Autodesk Fusion 360 part; units mm, degrees
(part 3 of 25)
  arc A722 (33.6042, 52.4764) -> (33.6042, 52.5272) centre (33.6042, 52.5018) ccw
  arc A723 (33.5788, 54.8259) -> (33.6296, 54.8259) centre (33.6042, 54.8259) ccw
  arc A724 (32.4358, 52.5272) -> (32.4358, 52.4764) centre (32.4358, 52.5018) ccw
  arc A725 (32.9297, 55.2154) -> (32.9805, 55.2154) centre (32.9551, 55.2154) ccw
  arc A726 (41.2242, 53.9821) -> (41.2242, 54.0329) centre (41.2242, 54.0075) ccw
  arc A727 (33.5788, 55.1504) -> (33.6296, 55.1504) centre (33.6042, 55.1504) ccw
  arc A728 (54.4034, 1.5804) -> (54.4542, 1.5804) centre (54.4288, 1.5804) ccw
  arc A729 (32.9297, 54.9557) -> (32.9805, 54.9557) centre (32.9551, 54.9557) ccw
  arc A730 (32.4104, 52.8264) -> (32.4612, 52.8264) centre (32.4358, 52.8264) ccw
  arc A731 (34.9758, 52.5272) -> (34.9758, 52.4764) centre (34.9758, 52.5018) ccw
  arc A732 (32.4612, 55.2154) -> (32.4104, 55.2154) centre (32.4358, 55.2154) ccw
  arc A733 (40.64, 54.8005) -> (40.64, 54.8513) centre (40.64, 54.8259) ccw
  arc A734 (29.7942, 28.6145) -> (29.7942, 28.6653) centre (29.7942, 28.6399) ccw
  arc A735 (32.7604, 53.1255) -> (32.7604, 53.1763) centre (32.7604, 53.1509) ccw
  arc A736 (32.6756, 53.667) -> (32.7153, 53.6988) centre (32.6955, 53.6829) ccw
  arc A737 (32.4358, 54.0329) -> (32.4358, 53.9821) centre (32.4358, 54.0075) ccw
  arc A738 (41.2496, 54.332) -> (41.1988, 54.332) centre (41.2242, 54.332) ccw
  arc A739 (40.0558, 55.1504) -> (40.2181, 54.9233) centre (40.2959, 55.1504) ccw
  arc A740 (33.6296, 52.8264) -> (33.5788, 52.8264) centre (33.6042, 52.8264) ccw
  line L231 (32.6954, 53.6829) -> (32.4358, 54.0075)
  arc A741 (40.2181, 54.9233) -> (40.64, 54.8259) centre (40.6401, 55.7886) ccw
  arc A742 (41.1988, 53.6829) -> (41.2496, 53.6829) centre (41.2242, 53.6829) ccw
  arc A743 (26.1112, 29.924) -> (26.0604, 29.924) centre (26.0858, 29.924) ccw
  arc A744 (32.7604, 53.1509) -> (32.4358, 52.8264) centre (32.7604, 52.8263) ccw
  arc A745 (33.6042, 52.8264) -> (33.2796, 53.1509) centre (33.2796, 52.8263) ccw
  arc A746 (40.2292, 54.9461) -> (40.2069, 54.9004) centre (40.2181, 54.9233) ccw
  arc A747 (33.6042, 53.9821) -> (33.6042, 54.0329) centre (33.6042, 54.0075) ccw
  arc A748 (32.9805, 55.2154) -> (32.9297, 55.2154) centre (32.9551, 55.2154) ccw
  arc A749 (33.5788, 53.6829) -> (33.6296, 53.6829) centre (33.6042, 53.6829) ccw
  line L232 (32.9551, 55.2154) -> (32.9551, 54.9557)
  line L233 (36.1442, 52.8264) -> (36.1442, 52.5018)
  line L234 (34.9758, 52.5018) -> (34.9758, 52.8264)
  arc A750 (36.1696, 52.8264) -> (36.1188, 52.8264) centre (36.1442, 52.8264) ccw
  arc A751 (36.1277, 54.8065) -> (36.1607, 54.8452) centre (36.1442, 54.8258) ccw
  arc A752 (37.8404, 53.1509) -> (37.5158, 52.8264) centre (37.8404, 52.8263) ccw
  arc A753 (36.1442, 52.8264) -> (35.8196, 53.1509) centre (35.8196, 52.8263) ccw
  arc A754 (34.9956, 54.0233) -> (34.956, 53.9916) centre (34.9758, 54.0074) ccw
  arc A755 (38.3596, 53.1763) -> (38.3596, 53.1255) centre (38.3596, 53.1509) ccw
  arc A756 (35.3004, 53.1509) -> (34.9758, 52.8264) centre (35.3004, 52.8263) ccw
  arc A757 (38.3596, 53.1255) -> (38.3596, 53.1763) centre (38.3596, 53.1509) ccw
  arc A758 (38.6842, 53.9821) -> (38.6842, 54.0329) centre (38.6842, 54.0075) ccw
  arc A759 (34.9504, 52.8264) -> (35.0012, 52.8264) centre (34.9758, 52.8264) ccw
  line L235 (35.4951, 55.3776) -> (36.1442, 54.8259)
  line L236 (37.7754, 54.8259) -> (37.5158, 55.1504)
  line L237 (35.3004, 53.1509) -> (35.8196, 53.1509)
  line L238 (37.5158, 52.5018) -> (37.5158, 52.8264)
  arc A760 (35.2679, 55.5004) -> (35.2679, 55.4496) centre (35.2679, 55.475) ccw
  arc A761 (36.1442, 53.9821) -> (36.1442, 54.0329) centre (36.1442, 54.0075) ccw
  arc A762 (37.5412, 52.8264) -> (37.4904, 52.8264) centre (37.5158, 52.8264) ccw
  line L239 (36.1442, 53.6829) -> (36.1442, 54.332)
  arc A763 (35.3004, 53.1763) -> (35.3004, 53.1255) centre (35.3004, 53.1509) ccw
  arc A764 (36.1188, 52.5018) -> (36.1696, 52.5018) centre (36.1442, 52.5018) ccw
  arc A765 (37.4904, 52.8264) -> (37.5412, 52.8264) centre (37.5158, 52.8264) ccw
  line L240 (38.6842, 52.8264) -> (38.6842, 52.5018)
  arc A766 (35.5115, 55.397) -> (35.4786, 55.3583) centre (35.495, 55.3777) ccw
  arc A767 (37.4904, 52.5018) -> (37.5412, 52.5018) centre (37.5158, 52.5018) ccw
  arc A768 (38.6588, 52.5018) -> (38.7096, 52.5018) centre (38.6842, 52.5018) ccw
  line L241 (37.5158, 54.0075) -> (38.6842, 54.0075)
  arc A769 (37.8404, 53.1255) -> (37.8404, 53.1763) centre (37.8404, 53.1509) ccw
  arc A770 (35.4951, 55.3776) -> (35.2679, 55.475) centre (35.2679, 55.1613) ccw
  line L242 (35.2354, 53.6829) -> (34.9758, 54.0075)
  arc A771 (38.6842, 52.4764) -> (38.6842, 52.5272) centre (38.6842, 52.5018) ccw
  arc A772 (37.8404, 53.1763) -> (37.8404, 53.1255) centre (37.8404, 53.1509) ccw
  arc A773 (35.8196, 53.1255) -> (35.8196, 53.1763) centre (35.8196, 53.1509) ccw
  arc A774 (36.1696, 54.332) -> (36.1188, 54.332) centre (36.1442, 54.332) ccw
  arc A775 (34.9504, 55.1829) -> (35.0012, 55.1829) centre (34.9758, 55.1829) ccw
  arc A776 (34.9758, 55.1829) -> (35.2354, 54.8259) centre (35.351, 55.1829) ccw
  arc A777 (34.9504, 52.5018) -> (35.0012, 52.5018) centre (34.9758, 52.5018) ccw
  line L243 (36.1442, 54.8259) -> (36.1442, 55.475)
  arc A778 (35.8196, 53.1763) -> (35.8196, 53.1255) centre (35.8196, 53.1509) ccw
  arc A779 (36.1188, 54.8259) -> (36.1696, 54.8259) centre (36.1442, 54.8259) ccw
  arc A780 (34.9758, 54.0329) -> (34.9758, 53.9821) centre (34.9758, 54.0075) ccw
  line L244 (34.9758, 54.0075) -> (36.1442, 54.0075)
  arc A781 (35.2679, 55.4496) -> (35.2679, 55.5004) centre (35.2679, 55.475) ccw
  arc A782 (36.1696, 55.475) -> (36.1188, 55.475) centre (36.1442, 55.475) ccw
  line L245 (38.6842, 52.5018) -> (37.5158, 52.5018)
  arc A783 (35.0012, 55.1829) -> (34.9504, 55.1829) centre (34.9758, 55.1829) ccw
  arc A784 (36.1188, 52.8264) -> (36.1696, 52.8264) centre (36.1442, 52.8264) ccw
  arc A785 (35.0012, 52.8264) -> (34.9504, 52.8264) centre (34.9758, 52.8264) ccw
  arc A786 (35.3004, 53.1255) -> (35.3004, 53.1763) centre (35.3004, 53.1509) ccw
  arc A787 (35.2679, 55.475) -> (34.9758, 55.1829) centre (35.2679, 55.1829) ccw
  arc A788 (35.4767, 55.3601) -> (35.5135, 55.3952) centre (35.4951, 55.3777) ccw
  arc A789 (37.5158, 52.5272) -> (37.5158, 52.4764) centre (37.5158, 52.5018) ccw
  arc A790 (36.1188, 53.6829) -> (36.1696, 53.6829) centre (36.1442, 53.6829) ccw
  line L246 (37.8404, 53.1509) -> (38.3596, 53.1509)
  arc A791 (38.7096, 52.8264) -> (38.6588, 52.8264) centre (38.6842, 52.8264) ccw
  arc A792 (38.6588, 52.8264) -> (38.7096, 52.8264) centre (38.6842, 52.8264) ccw
  arc A793 (38.6842, 52.8264) -> (38.3596, 53.1509) centre (38.3596, 52.8263) ccw
  arc A794 (37.5356, 54.0233) -> (37.496, 53.9916) centre (37.5158, 54.0074) ccw
  line L247 (37.7754, 53.6829) -> (37.5158, 54.0075)
  arc A795 (37.7556, 53.667) -> (37.7953, 53.6988) centre (37.7754, 53.6829) ccw
  arc A796 (35.2156, 53.667) -> (35.2553, 53.6988) centre (35.2355, 53.6829) ccw
  arc A797 (38.6588, 53.6829) -> (38.7096, 53.6829) centre (38.6842, 53.6829) ccw
  arc A798 (35.2276, 54.8017) -> (35.2433, 54.8501) centre (35.2355, 54.8259) ccw
  line L248 (37.5158, 55.1504) -> (38.6842, 55.1504)
  arc A799 (37.5158, 55.1758) -> (37.5158, 55.125) centre (37.5158, 55.1504) ccw
  arc A800 (38.7096, 54.332) -> (38.6588, 54.332) centre (38.6842, 54.332) ccw
  arc A801 (37.5356, 55.1663) -> (37.496, 55.1346) centre (37.5158, 55.1504) ccw
  arc A802 (37.7556, 54.81) -> (37.7953, 54.8418) centre (37.7754, 54.8259) ccw
  arc A803 (38.6842, 55.125) -> (38.6842, 55.1758) centre (38.6842, 55.1504) ccw
  line L249 (38.6842, 53.6829) -> (38.6842, 54.332)
  arc A804 (37.5158, 54.0329) -> (37.5158, 53.9821) centre (37.5158, 54.0075) ccw
  line L250 (41.2242, 52.5018) -> (40.0558, 52.5018)
  arc A805 (33.6804, 29.5557) -> (33.7312, 29.5557) centre (33.7058, 29.5557) ccw
  arc A806 (40.3804, 53.1255) -> (40.3804, 53.1763) centre (40.3804, 53.1509) ccw
  arc A807 (33.9979, 29.8478) -> (33.7058, 29.5557) centre (33.9979, 29.5557) ccw
  arc A808 (34.5567, 28.0882) -> (34.6075, 28.0882) centre (34.5821, 28.0882) ccw
  line L251 (38.6842, 54.8259) -> (38.6842, 55.475)
  line L252 (37.4974, 2.4892) -> (37.4974, 1.3208)
  arc A809 (38.6588, 54.8259) -> (38.7096, 54.8259) centre (38.6842, 54.8259) ccw
  arc A810 (40.0812, 52.8264) -> (40.0304, 52.8264) centre (40.0558, 52.8264) ccw
  arc A811 (41.2242, 52.4764) -> (41.2242, 52.5272) centre (41.2242, 52.5018) ccw
  arc A812 (40.3804, 53.1763) -> (40.3804, 53.1255) centre (40.3804, 53.1509) ccw
  line L253 (40.3804, 53.1509) -> (40.8996, 53.1509)
  line L254 (41.2242, 52.8264) -> (41.2242, 52.5018)
  arc A813 (34.6075, 28.6724) -> (34.5567, 28.6724) centre (34.5821, 28.6724) ccw
  arc A814 (40.0304, 52.8264) -> (40.0812, 52.8264) centre (40.0558, 52.8264) ccw
  arc A815 (40.3804, 53.1509) -> (40.0558, 52.8264) centre (40.3804, 52.8263) ccw
  arc A816 (41.2242, 52.8264) -> (40.8996, 53.1509) centre (40.8996, 52.8263) ccw
  arc A817 (37.157, 2.2494) -> (37.1888, 2.2097) centre (37.1729, 2.2296) ccw
  arc A818 (41.1988, 52.8264) -> (41.2496, 52.8264) centre (41.2242, 52.8264) ccw
  arc A819 (37.472, 1.3208) -> (37.5228, 1.3208) centre (37.4974, 1.3208) ccw
  line L255 (37.1729, 2.2296) -> (37.4974, 2.4892)
  arc A820 (37.1729, 1.3462) -> (37.1729, 1.2954) centre (37.1729, 1.3208) ccw
  line L256 (38.9636, 2.4892) -> (38.9636, 1.6454)
  arc A821 (34.8577, 29.1794) -> (34.8907, 29.2181) centre (34.8742, 29.1988) ccw
  arc A822 (37.5133, 2.4694) -> (37.4816, 2.509) centre (37.4975, 2.4892) ccw
  arc A823 (37.5228, 2.4892) -> (37.472, 2.4892) centre (37.4974, 2.4892) ccw
  line L257 (37.1729, 1.3208) -> (37.822, 1.3208)
  line L258 (40.0558, 52.5018) -> (40.0558, 52.8264)
  arc A824 (40.0304, 52.5018) -> (40.0812, 52.5018) centre (40.0558, 52.5018) ccw
  arc A825 (40.8996, 53.1763) -> (40.8996, 53.1255) centre (40.8996, 53.1509) ccw
  arc A826 (40.0558, 52.5272) -> (40.0558, 52.4764) centre (40.0558, 52.5018) ccw
  arc A827 (38.7096, 55.475) -> (38.6588, 55.475) centre (38.6842, 55.475) ccw
  arc A828 (40.8996, 53.1255) -> (40.8996, 53.1763) centre (40.8996, 53.1509) ccw
  arc A829 (33.9979, 29.8732) -> (33.9979, 29.8224) centre (33.9979, 29.8478) ccw
  arc A830 (38.9382, 1.6454) -> (38.989, 1.6454) centre (38.9636, 1.6454) ccw
  arc A831 (39.6381, 2.4892) -> (39.5873, 2.4892) centre (39.6127, 2.4892) ccw
  line L259 (39.6127, 1.6454) -> (39.6127, 2.4892)
  line L260 (44.8779, 1.3208) -> (44.6182, 1.8401)
  arc A832 (41.33, 2.5146) -> (41.33, 2.4638) centre (41.33, 2.4892) ccw
  arc A833 (45.3263, 1.4831) -> (45.7157, 1.3208) centre (45.7158, 1.8692) ccw
  arc A834 (41.5897, 2.4638) -> (41.5897, 2.5146) centre (41.5897, 2.4892) ccw
  line L261 (41.4598, 2.4892) -> (41.4598, 1.3208)
  line L262 (41.33, 2.4892) -> (41.5897, 2.4892)
  arc A835 (41.33, 1.3462) -> (41.33, 1.2954) centre (41.33, 1.3208) ccw
  arc A836 (40.2082, 2.4892) -> (40.1574, 2.4892) centre (40.1828, 2.4892) ccw
  arc A837 (37.822, 1.2954) -> (37.822, 1.3462) centre (37.822, 1.3208) ccw
  arc A838 (40.1574, 1.3208) -> (40.2082, 1.3208) centre (40.1828, 1.3208) ccw
  arc A839 (40.8065, 1.3208) -> (40.8573, 1.3208) centre (40.8319, 1.3208) ccw
  line L263 (42.3742, 1.3208) -> (42.7637, 2.4892)
  line L264 (43.233, 2.4892) -> (43.7523, 2.4892)
  line L265 (43.7523, 1.3208) -> (43.233, 1.3208)
  arc A840 (42.3501, 1.3288) -> (42.3983, 1.3128) centre (42.3742, 1.3208) ccw
  arc A841 (43.6225, 1.9445) -> (43.6225, 1.9953) centre (43.6225, 1.9699) ccw
  arc A842 (44.2033, 1.3208) -> (44.2541, 1.3208) centre (44.2287, 1.3208) ccw
  arc A843 (44.2287, 2.5146) -> (44.2287, 2.4638) centre (44.2287, 2.4892) ccw
  arc A844 (41.4852, 2.4892) -> (41.4344, 2.4892) centre (41.4598, 2.4892) ccw
  line L266 (41.9848, 2.4892) -> (42.3742, 1.3208)
  line L267 (40.1828, 2.4892) -> (40.8319, 1.3208)
  arc A845 (38.9636, 1.6454) -> (39.6127, 1.6454) centre (39.2881, 1.6454) ccw
  arc A846 (40.8097, 1.3085) -> (40.8541, 1.3331) centre (40.8319, 1.3208) ccw
  arc A847 (40.205, 2.5015) -> (40.1606, 2.4769) centre (40.1828, 2.4892) ccw
  arc A848 (40.8573, 2.4892) -> (40.8065, 2.4892) centre (40.8319, 2.4892) ccw
  arc A849 (44.5533, 1.8655) -> (44.5533, 1.8147) centre (44.5533, 1.8401) ccw
  arc A850 (43.233, 1.3462) -> (43.233, 1.2954) centre (43.233, 1.3208) ccw
  line L268 (44.5533, 1.8401) -> (44.2287, 1.8401)
  arc A851 (44.8551, 1.3094) -> (44.9006, 1.3322) centre (44.8779, 1.3208) ccw
  arc A852 (43.7523, 1.2954) -> (43.7523, 1.3462) centre (43.7523, 1.3208) ccw
  arc A853 (43.2076, 1.3208) -> (43.2584, 1.3208) centre (43.233, 1.3208) ccw
  arc A854 (41.4344, 1.3208) -> (41.4852, 1.3208) centre (41.4598, 1.3208) ccw
  arc A855 (38.989, 1.6454) -> (38.9382, 1.6454) centre (38.9636, 1.6454) ccw
  arc A856 (42.7878, 2.4812) -> (42.7396, 2.4972) centre (42.7637, 2.4892) ccw
  arc A857 (39.6381, 1.6454) -> (39.5873, 1.6454) centre (39.6127, 1.6454) ccw
  arc A858 (39.5873, 1.6454) -> (39.6381, 1.6454) centre (39.6127, 1.6454) ccw
  line L269 (40.1828, 1.3208) -> (40.1828, 2.4892)
  line L270 (41.33, 1.3208) -> (41.5897, 1.3208)
  line L271 (40.8319, 1.3208) -> (40.8319, 2.4892)
  arc A859 (42.0089, 2.4972) -> (41.9607, 2.4812) centre (41.9848, 2.4892) ccw
  arc A860 (43.7523, 2.4638) -> (43.7523, 2.5146) centre (43.7523, 2.4892) ccw
  arc A861 (43.233, 2.5146) -> (43.233, 2.4638) centre (43.233, 2.4892) ccw
  arc A862 (43.233, 1.9953) -> (43.233, 1.9445) centre (43.233, 1.9699) ccw
  line L272 (44.2287, 1.3208) -> (44.2287, 2.4892)
  arc A863 (44.5533, 2.4638) -> (44.5533, 2.5146) centre (44.5533, 2.4892) ccw
  arc A864 (42.3501, 1.3128) -> (42.3983, 1.3288) centre (42.3742, 1.3208) ccw
  line L273 (43.233, 1.3208) -> (43.233, 2.4892)
  arc A865 (44.2541, 2.4892) -> (44.2033, 2.4892) centre (44.2287, 2.4892) ccw
  line L274 (43.233, 1.9699) -> (43.6225, 1.9699)
  arc A866 (44.5533, 2.5146) -> (44.5533, 2.4638) centre (44.5533, 2.4892) ccw
  arc A867 (44.5533, 1.8401) -> (44.5533, 2.4892) centre (44.5533, 2.1646) ccw
  arc A868 (43.2584, 2.4892) -> (43.2076, 2.4892) centre (43.233, 2.4892) ccw
  arc A869 (38.989, 2.4892) -> (38.9382, 2.4892) centre (38.9636, 2.4892) ccw
  arc A870 (41.5897, 1.2954) -> (41.5897, 1.3462) centre (41.5897, 1.3208) ccw
  arc A871 (44.6409, 1.8514) -> (44.5955, 1.8287) centre (44.6182, 1.8401) ccw
  arc A872 (44.5533, 1.8147) -> (44.5533, 1.8655) centre (44.5533, 1.8401) ccw
  arc A873 (44.2287, 1.8655) -> (44.2287, 1.8147) centre (44.2287, 1.8401) ccw
  arc A874 (45.7157, 1.3462) -> (45.7157, 1.2954) centre (45.7157, 1.3208) ccw
  line L275 (44.2287, 2.4892) -> (44.5533, 2.4892)
  arc A875 (49.554, 1.8401) -> (49.554, 2.4892) centre (49.554, 2.1646) ccw
  arc A876 (47.6145, 1.3462) -> (47.6145, 1.2954) centre (47.6145, 1.3208) ccw
  arc A877 (50.6874, 2.4638) -> (50.6874, 2.5146) centre (50.6874, 2.4892) ccw
  arc A878 (52.1222, 2.1646) -> (52.173, 2.1646) centre (52.1476, 2.1646) ccw
  line L276 (45.8456, 1.8076) -> (45.4886, 2.0024)
  arc A879 (47.6399, 2.4892) -> (47.5891, 2.4892) centre (47.6145, 2.4892) ccw
  arc A880 (49.554, 2.5146) -> (49.554, 2.4638) centre (49.554, 2.4892) ccw
  arc A881 (45.6184, 2.5146) -> (45.6184, 2.4638) centre (45.6184, 2.4892) ccw
  arc A882 (49.204, 1.3208) -> (49.2548, 1.3208) centre (49.2294, 1.3208) ccw
  arc A883 (45.6184, 2.4892) -> (45.3587, 2.2296) centre (45.6184, 2.2295) ccw
  line L277 (49.554, 1.8401) -> (49.2294, 1.8401)
  arc A884 (49.2548, 2.4892) -> (49.204, 2.4892) centre (49.2294, 2.4892) ccw
  arc A885 (50.6874, 1.8147) -> (50.6874, 1.8655) centre (50.6874, 1.8401) ccw
  line L278 (46.7557, 2.4892) -> (47.1452, 1.3208)
  arc A886 (45.7157, 1.2954) -> (45.7157, 1.3462) centre (45.7157, 1.3208) ccw
  arc A887 (45.9105, 2.3918) -> (45.6184, 2.4892) centre (45.6184, 2.0024) ccw
  arc A888 (45.3841, 2.2296) -> (45.3333, 2.2296) centre (45.3587, 2.2296) ccw
  arc A889 (47.5891, 1.3208) -> (47.6399, 1.3208) centre (47.6145, 1.3208) ccw
  line L279 (47.6145, 1.3208) -> (48.1338, 1.3208)
  line L280 (49.2294, 2.4892) -> (49.554, 2.4892)
  arc A890 (49.554, 2.4638) -> (49.554, 2.5146) centre (49.554, 2.4892) ccw
  arc A891 (49.554, 1.8147) -> (49.554, 1.8655) centre (49.554, 1.8401) ccw
  arc A892 (45.8585, 1.8295) -> (45.8327, 1.7857) centre (45.8456, 1.8076) ccw
  arc A893 (45.3587, 2.2296) -> (45.4886, 2.0024) centre (45.6224, 2.2296) ccw
  arc A894 (45.5007, 2.0247) -> (45.4764, 1.9801) centre (45.4886, 2.0024) ccw
  arc A895 (46.0008, 1.5804) -> (45.95, 1.5804) centre (45.9754, 1.5804) ccw
  arc A896 (46.4636, 1.6383) -> (46.4636, 1.5875) centre (46.4636, 1.6129) ccw
  arc A897 (50.3374, 1.3208) -> (50.3882, 1.3208) centre (50.3628, 1.3208) ccw
  arc A898 (45.7157, 1.3208) -> (45.9754, 1.5804) centre (45.7157, 1.5805) ccw
  arc A899 (45.3333, 2.2296) -> (45.3841, 2.2296) centre (45.3587, 2.2296) ccw
  arc A900 (45.8334, 1.7853) -> (45.8577, 1.8299) centre (45.8455, 1.8076) ccw
  arc A901 (50.3628, 2.5146) -> (50.3628, 2.4638) centre (50.3628, 2.4892) ccw
  line L281 (50.6874, 1.8401) -> (50.3628, 1.8401)
  arc A902 (49.2294, 2.5146) -> (49.2294, 2.4638) centre (49.2294, 2.4892) ccw
  arc A903 (50.6874, 1.8655) -> (50.6874, 1.8147) centre (50.6874, 1.8401) ccw
  arc A904 (50.3628, 1.8655) -> (50.3628, 1.8147) centre (50.3628, 1.8401) ccw
  arc A905 (50.775, 1.8514) -> (50.7296, 1.8287) centre (50.7523, 1.8401) ccw
  arc A906 (48.1338, 1.2954) -> (48.1338, 1.3462) centre (48.1338, 1.3208) ccw
  arc A907 (45.6184, 2.4638) -> (45.6184, 2.5146) centre (45.6184, 2.4892) ccw
  arc A908 (46.3422, 1.3288) -> (46.3904, 1.3128) centre (46.3663, 1.3208) ccw
  arc A909 (45.95, 1.5804) -> (46.0008, 1.5804) centre (45.9754, 1.5804) ccw
  arc A910 (47.1211, 1.3128) -> (47.1693, 1.3288) centre (47.1452, 1.3208) ccw
  line L282 (50.3628, 1.3208) -> (50.3628, 2.4892)
  line L283 (50.3628, 2.4892) -> (50.6874, 2.4892)
  arc A911 (50.3882, 2.4892) -> (50.3374, 2.4892) centre (50.3628, 2.4892) ccw
  line L284 (51.0119, 1.3208) -> (50.7523, 1.8401)
  arc A912 (45.9754, 1.5804) -> (45.8456, 1.8076) centre (45.7117, 1.5804) ccw
  arc A913 (46.7798, 2.4972) -> (46.7316, 2.4812) centre (46.7557, 2.4892) ccw
  arc A914 (45.4757, 1.9805) -> (45.5014, 2.0242) centre (45.4885, 2.0024) ccw
  line L285 (47.0478, 1.6129) -> (46.4636, 1.6129)
  line L286 (47.6145, 2.4892) -> (47.6145, 1.3208)
  line L287 (49.2294, 1.3208) -> (49.2294, 2.4892)
  arc A915 (49.554, 1.8655) -> (49.554, 1.8147) centre (49.554, 1.8401) ccw
  line L288 (51.4985, 1.6454) -> (51.4985, 2.1646)
  arc A916 (52.1476, 2.1646) -> (51.4985, 2.1646) centre (51.8231, 2.1646) ccw
  arc A917 (50.6874, 1.8401) -> (50.6874, 2.4892) centre (50.6874, 2.1646) ccw
  line L289 (46.3663, 1.3208) -> (46.7557, 2.4892)
  arc A918 (45.8952, 2.3715) -> (45.9257, 2.4122) centre (45.9105, 2.3918) ccw
  arc A919 (46.7798, 2.4812) -> (46.7316, 2.4972) centre (46.7557, 2.4892) ccw
  arc A920 (47.0478, 1.5875) -> (47.0478, 1.6383) centre (47.0478, 1.6129) ccw
  arc A921 (50.6874, 2.5146) -> (50.6874, 2.4638) centre (50.6874, 2.4892) ccw
  arc A922 (49.2294, 1.8655) -> (49.2294, 1.8147) centre (49.2294, 1.8401) ccw
  arc A923 (50.9892, 1.3094) -> (51.0347, 1.3322) centre (51.0119, 1.3208) ccw
  arc A924 (45.3443, 1.501) -> (45.3082, 1.4652) centre (45.3262, 1.4831) ccw
  arc A925 (27.4884, 51.9684) -> (27.4884, 52.0192) centre (27.4884, 51.9938) ccw
  arc A926 (27.2542, 52.6429) -> (27.2034, 52.6429) centre (27.2288, 52.6429) ccw
  arc A927 (52.6546, 1.3462) -> (52.6546, 1.2954) centre (52.6546, 1.3208) ccw
  arc A928 (52.8888, 1.5804) -> (52.9396, 1.5804) centre (52.9142, 1.5804) ccw
  arc A929 (50.2412, 29.924) -> (50.1904, 29.924) centre (50.2158, 29.924) ccw
  line L290 (50.7351, 29.6644) -> (50.7351, 29.2749)
  line L291 (52.6546, 1.3208) -> (52.5248, 1.3208)
  arc A930 (50.2238, 31.156) -> (50.2078, 31.1078) centre (50.2158, 31.1319) ccw
  arc A931 (27.7227, 52.4482) -> (27.7735, 52.4482) centre (27.7481, 52.4482) ccw
  arc A932 (52.173, 1.6454) -> (52.1222, 1.6454) centre (52.1476, 1.6454) ccw
  line L292 (53.4819, 1.9699) -> (53.8714, 1.9699)
  arc A933 (51.5239, 2.1646) -> (51.4731, 2.1646) centre (51.4985, 2.1646) ccw
  arc A934 (52.9396, 2.4892) -> (52.8888, 2.4892) centre (52.9142, 2.4892) ccw
  line L293 (52.9142, 2.4892) -> (52.9142, 1.5804)
  arc A935 (51.5239, 1.6454) -> (51.4731, 1.6454) centre (51.4985, 1.6454) ccw
  arc A936 (54.0012, 1.2954) -> (54.0012, 1.3462) centre (54.0012, 1.3208) ccw
  arc A937 (50.7097, 29.6644) -> (50.7605, 29.6644) centre (50.7351, 29.6644) ccw
  arc A938 (27.7735, 52.6429) -> (27.7227, 52.6429) centre (27.7481, 52.6429) ccw
  arc A939 (51.4985, 1.6454) -> (52.1476, 1.6454) centre (51.8231, 1.6454) ccw
  line L294 (50.2158, 30.353) -> (51.3842, 30.7425)
  arc A940 (28.3972, 52.6175) -> (28.3972, 52.6683) centre (28.3972, 52.6429) ccw
  arc A941 (27.7481, 52.6683) -> (27.7481, 52.6175) centre (27.7481, 52.6429) ccw
  line L295 (27.7481, 52.4482) -> (27.7481, 52.6429)
  line L296 (28.3972, 52.6429) -> (28.3972, 52.2534)
  arc A942 (52.6546, 1.3208) -> (52.9142, 1.5804) centre (52.6546, 1.5804) ccw
  line L297 (54.0012, 1.3208) -> (53.4819, 1.3208)
  line L298 (51.3842, 30.7425) -> (50.2158, 31.1319)
  arc A943 (51.3762, 30.7184) -> (51.3922, 30.7666) centre (51.3842, 30.7425) ccw
  line L299 (53.4819, 1.3208) -> (53.4819, 2.4892)
  arc A944 (50.7605, 29.6644) -> (50.7097, 29.6644) centre (50.7351, 29.6644) ccw
  arc A945 (28.1376, 52.0192) -> (28.1376, 51.9684) centre (28.1376, 51.9938) ccw
  arc A946 (50.2158, 29.3003) -> (50.2158, 29.2495) centre (50.2158, 29.2749) ccw
  line L300 (50.2158, 29.2749) -> (50.2158, 29.924)
  arc A947 (28.4226, 52.2534) -> (28.3718, 52.2534) centre (28.3972, 52.2534) ccw
  line L301 (28.1376, 51.9938) -> (27.4884, 51.9938)
  arc A948 (27.4884, 52.0192) -> (27.4884, 51.9684) centre (27.4884, 51.9938) ccw
  arc A949 (50.7097, 29.2749) -> (50.7605, 29.2749) centre (50.7351, 29.2749) ccw
  arc A950 (53.4565, 1.3208) -> (53.5073, 1.3208) centre (53.4819, 1.3208) ccw
  arc A951 (28.1376, 51.9684) -> (28.1376, 52.0192) centre (28.1376, 51.9938) ccw
  arc A952 (52.1222, 1.6454) -> (52.173, 1.6454) centre (52.1476, 1.6454) ccw
  arc A953 (52.9396, 1.5804) -> (52.8888, 1.5804) centre (52.9142, 1.5804) ccw
  arc A954 (28.3718, 52.2534) -> (28.4226, 52.2534) centre (28.3972, 52.2534) ccw
  arc A955 (36.0299, 1.3462) -> (36.0299, 1.2954) centre (36.0299, 1.3208) ccw
  line L302 (53.4819, 2.4892) -> (54.0012, 2.4892)
  arc A956 (28.1376, 51.9938) -> (28.3972, 52.2534) centre (28.1376, 52.2534) ccw
  arc A957 (27.2288, 52.2534) -> (27.4884, 51.9938) centre (27.4884, 52.2534) ccw
  line L303 (52.1476, 2.1646) -> (52.1476, 1.6454)
  arc A958 (50.7351, 29.2495) -> (50.7351, 29.3003) centre (50.7351, 29.2749) ccw
  arc A959 (52.173, 2.1646) -> (52.1222, 2.1646) centre (52.1476, 2.1646) ccw
  arc A960 (54.6885, 1.3462) -> (54.6885, 1.2954) centre (54.6885, 1.3208) ccw
  arc A961 (50.1904, 29.2749) -> (50.2412, 29.2749) centre (50.2158, 29.2749) ccw
  arc A962 (50.2078, 30.3771) -> (50.2238, 30.3289) centre (50.2158, 30.353) ccw
  arc A963 (51.4731, 1.6454) -> (51.5239, 1.6454) centre (51.4985, 1.6454) ccw
  arc A964 (51.3922, 30.7184) -> (51.3762, 30.7666) centre (51.3842, 30.7425) ccw
  line L304 (50.7351, 29.2749) -> (50.2158, 29.2749)
  arc A965 (52.5248, 1.3462) -> (52.5248, 1.2954) centre (52.5248, 1.3208) ccw
  arc A966 (54.0012, 2.4638) -> (54.0012, 2.5146) centre (54.0012, 2.4892) ccw
  arc A967 (28.4226, 52.6429) -> (28.3718, 52.6429) centre (28.3972, 52.6429) ccw
  arc A968 (53.4819, 1.3462) -> (53.4819, 1.2954) centre (53.4819, 1.3208) ccw
  line L305 (27.7481, 52.6429) -> (28.3972, 52.6429)
  arc A969 (51.4731, 2.1646) -> (51.5239, 2.1646) centre (51.4985, 2.1646) ccw
  arc A970 (53.5073, 2.4892) -> (53.4565, 2.4892) centre (53.4819, 2.4892) ccw
  arc A971 (52.6546, 1.2954) -> (52.6546, 1.3462) centre (52.6546, 1.3208) ccw
  arc A972 (27.2542, 52.2534) -> (27.2034, 52.2534) centre (27.2288, 52.2534) ccw
  arc A973 (64.08, 47.4274) -> (64.1562, 47.4274) centre (64.1181, 47.4274) ccw
  arc A974 (28.1968, 7.6581) -> (28.1968, 7.7343) centre (28.1968, 7.6962) ccw
  line L306 (28.3972, 54.7567) -> (28.3972, 54.4322)
  arc A975 (28.1968, 7.6962) -> (28.5581, 8.0574) centre (28.1968, 8.0575) ccw
  arc A976 (28.0162, 7.7343) -> (28.0162, 7.6581) centre (28.0162, 7.6962) ccw
  arc A977 (27.5534, 55.1067) -> (27.5534, 55.0559) centre (27.5534, 55.0813) ccw
  line L307 (29.7163, 9.3218) -> (29.7163, 7.6962)
  arc A978 (29.6782, 7.6962) -> (29.7544, 7.6962) centre (29.7163, 7.6962) ccw
  arc A979 (29.2648, 7.7343) -> (29.2648, 7.6581) centre (29.2648, 7.6962) ccw
  arc A980 (27.2034, 54.4322) -> (27.2542, 54.4322) centre (27.2288, 54.4322) ccw
  arc A981 (29.7544, 9.3218) -> (29.6782, 9.3218) centre (29.7163, 9.3218) ccw
  arc A982 (27.5534, 55.0813) -> (27.2288, 54.7567) centre (27.5534, 54.7567) ccw
  line L308 (27.5534, 55.0813) -> (28.0726, 55.0813)
  line L309 (64.1181, 48.6918) -> (64.1181, 47.4274)
  arc A983 (65.7279, 48.2854) -> (65.3215, 48.6918) centre (65.3215, 48.2854) ccw
  arc A984 (63.7568, 47.0281) -> (63.7568, 47.1043) centre (63.7568, 47.0662) ccw
  line L310 (28.3972, 54.4322) -> (27.2288, 54.4322)
  arc A985 (63.5762, 47.1043) -> (63.5762, 47.0281) centre (63.5762, 47.0662) ccw
  line L311 (28.5581, 9.3218) -> (28.5581, 8.0574)
  line L312 (28.3972, 53.213) -> (27.2288, 53.213)
  arc A986 (65.3215, 48.7299) -> (65.3215, 48.6537) centre (65.3215, 48.6918) ccw
  arc A987 (65.3215, 48.6537) -> (65.3215, 48.7299) centre (65.3215, 48.6918) ccw
  arc A988 (64.7885, 48.3423) -> (64.861, 48.3188) centre (64.8248, 48.3306) ccw
  arc A989 (65.5661, 47.9969) -> (65.6187, 47.9417) centre (65.5924, 47.9693) ccw
  arc A990 (28.1968, 7.7343) -> (28.1968, 7.6581) centre (28.1968, 7.6962) ccw
  arc A991 (28.5962, 8.0574) -> (28.52, 8.0574) centre (28.5581, 8.0574) ccw
  arc A992 (63.7568, 47.0662) -> (64.1181, 47.4274) centre (63.7568, 47.4275) ccw
  arc A993 (65.3215, 48.6918) -> (64.8248, 48.3306) centre (65.3215, 48.1697) ccw
  arc A994 (65.5924, 47.9693) -> (65.7279, 48.2854) centre (65.2914, 48.2854) ccw
  arc A995 (28.3972, 54.4068) -> (28.3972, 54.4576) centre (28.3972, 54.4322) ccw
  arc A996 (27.2034, 54.7567) -> (27.2542, 54.7567) centre (27.2288, 54.7567) ccw
  arc A997 (28.3718, 54.4322) -> (28.4226, 54.4322) centre (28.3972, 54.4322) ccw
  arc A998 (28.4226, 54.7567) -> (28.3718, 54.7567) centre (28.3972, 54.7567) ccw
  line L313 (27.2288, 53.213) -> (28.3972, 53.8621)
  arc A999 (27.2034, 52.2534) -> (27.2542, 52.2534) centre (27.2288, 52.2534) ccw
  line L314 (28.3972, 53.8621) -> (27.2288, 53.8621)
  arc A1000 (28.3972, 54.7567) -> (28.0726, 55.0813) centre (28.0726, 54.7567) ccw
  line L315 (27.2288, 54.4322) -> (27.2288, 54.7567)
  arc A1001 (29.241, 8.9903) -> (29.2886, 8.9308) centre (29.2648, 8.9605) ccw
  arc A1002 (63.7568, 47.1043) -> (63.7568, 47.0281) centre (63.7568, 47.0662) ccw
  line L316 (29.2648, 7.6962) -> (30.1679, 7.6962)
  arc A1003 (28.4095, 53.8399) -> (28.3849, 53.8843) centre (28.3972, 53.8621) ccw
  arc A1004 (27.2542, 54.7567) -> (27.2034, 54.7567) centre (27.2288, 54.7567) ccw
  arc A1005 (27.5534, 55.0559) -> (27.5534, 55.1067) centre (27.5534, 55.0813) ccw
  line L317 (28.1968, 7.6962) -> (28.0162, 7.6962)
  arc A1006 (64.1562, 47.4274) -> (64.08, 47.4274) centre (64.1181, 47.4274) ccw
  arc A1007 (27.2288, 54.4576) -> (27.2288, 54.4068) centre (27.2288, 54.4322) ccw
  arc A1008 (28.3972, 53.1876) -> (28.3972, 53.2384) centre (28.3972, 53.213) ccw
  arc A1009 (28.0726, 55.1067) -> (28.0726, 55.0559) centre (28.0726, 55.0813) ccw
  arc A1010 (28.5962, 9.3218) -> (28.52, 9.3218) centre (28.5581, 9.3218) ccw
  arc A1011 (27.2288, 53.2384) -> (27.2288, 53.1876) centre (27.2288, 53.213) ccw
  arc A1012 (28.3972, 53.8367) -> (28.3972, 53.8875) centre (28.3972, 53.8621) ccw
  arc A1013 (28.3718, 54.7567) -> (28.4226, 54.7567) centre (28.3972, 54.7567) ccw
  arc A1014 (27.2165, 53.2352) -> (27.2411, 53.1908) centre (27.2288, 53.213) ccw
  arc A1015 (28.0726, 55.0559) -> (28.0726, 55.1067) centre (28.0726, 55.0813) ccw
  arc A1016 (28.52, 8.0574) -> (28.5962, 8.0574) centre (28.5581, 8.0574) ccw
  line L318 (27.2288, 52.2534) -> (27.2288, 52.6429)
  arc A1017 (29.7401, 9.292) -> (29.6925, 9.3516) centre (29.7163, 9.3218) ccw
  line L319 (29.2648, 8.9606) -> (29.7163, 9.3218)
  arc A1018 (30.1679, 7.6581) -> (30.1679, 7.7343) centre (30.1679, 7.6962) ccw
  arc A1019 (64.1562, 48.6918) -> (64.08, 48.6918) centre (64.1181, 48.6918) ccw
  line L320 (63.7568, 47.0662) -> (63.5762, 47.0662)
  arc A1020 (65.6898, 48.2854) -> (65.766, 48.2854) centre (65.7279, 48.2854) ccw
  arc A1021 (27.2288, 53.8875) -> (27.2288, 53.8367) centre (27.2288, 53.8621) ccw
  arc A1022 (31.8008, 2.5146) -> (31.8008, 2.4638) centre (31.8008, 2.4892) ccw
  arc A1023 (65.6214, 47.9446) -> (65.5634, 47.994) centre (65.5924, 47.9693) ccw
  arc A1024 (33.504, 1.5804) -> (33.4532, 1.5804) centre (33.4786, 1.5804) ccw
  arc A1025 (34.1907, 2.4638) -> (34.1907, 2.5146) centre (34.1907, 2.4892) ccw
  arc A1026 (34.4504, 2.4638) -> (34.4504, 2.5146) centre (34.4504, 2.4892) ccw
  arc A1027 (32.4499, 2.4638) -> (32.4499, 2.5146) centre (32.4499, 2.4892) ccw
  arc A1028 (33.219, 1.3462) -> (33.219, 1.2954) centre (33.219, 1.3208) ccw
  arc A1029 (33.4532, 1.5804) -> (33.504, 1.5804) centre (33.4786, 1.5804) ccw
  arc A1030 (65.766, 48.2854) -> (65.6898, 48.2854) centre (65.7279, 48.2854) ccw
  arc A1031 (65.7279, 47.0281) -> (65.7279, 47.1043) centre (65.7279, 47.0662) ccw
  arc A1032 (32.8873, 2.2296) -> (32.8366, 2.2296) centre (32.862, 2.2296) ccw
  line L321 (64.8248, 47.0662) -> (65.7279, 47.0662)
  arc A1033 (33.3366, 1.7853) -> (33.3609, 1.8299) centre (33.3488, 1.8076) ccw
  line L322 (34.4504, 1.3208) -> (34.1907, 1.3208)
  arc A1034 (64.8248, 47.1043) -> (64.8248, 47.0281) centre (64.8248, 47.0662) ccw
  arc A1035 (33.9565, 2.2296) -> (33.9057, 2.2296) centre (33.9311, 2.2296) ccw
  arc A1036 (32.9789, 1.9805) -> (33.0047, 2.0242) centre (32.9918, 2.0023) ccw
  arc A1037 (33.1216, 2.4892) -> (32.862, 2.2296) centre (33.1216, 2.2296) ccw
  arc A1038 (33.4786, 1.5804) -> (33.3488, 1.8076) centre (33.2149, 1.5804) ccw
  arc A1039 (34.1907, 1.2954) -> (34.1907, 1.3462) centre (34.1907, 1.3208) ccw
  arc A1040 (32.1, 1.3208) -> (32.1508, 1.3208) centre (32.1254, 1.3208) ccw
  arc A1041 (33.219, 1.2954) -> (33.219, 1.3462) centre (33.219, 1.3208) ccw
  arc A1042 (33.1216, 2.5146) -> (33.1216, 2.4638) centre (33.1216, 2.4892) ccw
  arc A1043 (33.9057, 1.5804) -> (33.9565, 1.5804) centre (33.9311, 1.5804) ccw
  arc A1044 (33.9057, 2.2296) -> (33.9565, 2.2296) centre (33.9311, 2.2296) ccw
  arc A1045 (34.1907, 2.4892) -> (33.9311, 2.2296) centre (34.1907, 2.2296) ccw
  line L323 (34.1907, 2.4892) -> (34.4504, 2.4892)
  arc A1046 (34.871, 2.2494) -> (34.9028, 2.2097) centre (34.8869, 2.2295) ccw
  line L324 (34.8869, 2.2296) -> (35.2114, 2.4892)
  arc A1047 (35.2368, 2.4892) -> (35.186, 2.4892) centre (35.2114, 2.4892) ccw
  arc A1048 (32.8475, 1.501) -> (32.8115, 1.4652) centre (32.8295, 1.4831) ccw
  arc A1049 (32.8366, 2.2296) -> (32.8873, 2.2296) centre (32.862, 2.2296) ccw
  arc A1050 (34.8869, 1.3462) -> (34.8869, 1.2954) centre (34.8869, 1.3208) ccw
  line L325 (32.1254, 1.3208) -> (32.1254, 2.4892)
  line L326 (36.0299, 2.2296) -> (36.3544, 2.4892)
  line L327 (65.5924, 47.9693) -> (64.8248, 47.0662)
  line L328 (34.8869, 1.3208) -> (35.536, 1.3208)
  arc A1051 (36.3703, 2.4694) -> (36.3386, 2.509) centre (36.3544, 2.4892) ccw
  arc A1052 (36.014, 2.2494) -> (36.0458, 2.2097) centre (36.0299, 2.2295) ccw
  line L329 (31.8008, 2.4892) -> (32.4499, 2.4892)
  arc A1053 (33.9311, 1.5804) -> (34.1907, 1.3208) centre (34.1907, 1.5804) ccw
  arc A1054 (33.1216, 2.4638) -> (33.1216, 2.5146) centre (33.1216, 2.4892) ccw
  arc A1055 (33.3985, 2.3715) -> (33.4289, 2.4122) centre (33.4137, 2.3918) ccw
  line L330 (33.3488, 1.8076) -> (32.9918, 2.0024)
  arc A1056 (35.2273, 2.4694) -> (35.1956, 2.509) centre (35.2114, 2.4892) ccw
  line L331 (36.3544, 2.4892) -> (36.3544, 1.3208)
  arc A1057 (34.4504, 1.2954) -> (34.4504, 1.3462) centre (34.4504, 1.3208) ccw
  arc A1058 (33.219, 1.3208) -> (33.4786, 1.5804) centre (33.219, 1.5804) ccw
  arc A1059 (64.7957, 47.0909) -> (64.8538, 47.0415) centre (64.8247, 47.0662) ccw
  arc A1060 (32.1508, 2.4892) -> (32.1, 2.4892) centre (32.1254, 2.4892) ccw
  line L332 (33.9311, 1.5804) -> (33.9311, 2.2296)
  arc A1061 (53.8714, 1.9445) -> (53.8714, 1.9953) centre (53.8714, 1.9699) ccw
  arc A1062 (34.1907, 1.3462) -> (34.1907, 1.2954) centre (34.1907, 1.3208) ccw
  line L333 (54.9481, 1.3208) -> (54.6885, 1.3208)
  arc A1063 (33.0039, 2.0247) -> (32.9796, 1.9801) centre (32.9917, 2.0024) ccw
  arc A1064 (33.4137, 2.3918) -> (33.1216, 2.4892) centre (33.1216, 2.0024) ccw
  arc A1065 (34.1907, 2.5146) -> (34.1907, 2.4638) centre (34.1907, 2.4892) ccw
  arc A1066 (35.186, 1.3208) -> (35.2368, 1.3208) centre (35.2114, 1.3208) ccw
  arc A1067 (35.536, 1.2954) -> (35.536, 1.3462) centre (35.536, 1.3208) ccw
  arc A1068 (32.862, 2.2296) -> (32.9918, 2.0024) centre (33.1257, 2.2296) ccw
  arc A1069 (33.3617, 1.8295) -> (33.3359, 1.7857) centre (33.3488, 1.8076) ccw
  arc A1070 (32.8295, 1.4831) -> (33.219, 1.3208) centre (33.219, 1.8694) ccw
  arc A1071 (33.9565, 1.5804) -> (33.9057, 1.5804) centre (33.9311, 1.5804) ccw
  line L334 (35.2114, 2.4892) -> (35.2114, 1.3208)
  line L335 (59.134, 11.2155) -> (57.706, 11.7348)
  line L336 (34.2251, 29.7505) -> (34.8742, 29.1987)
  arc A1072 (33.9576, 29.1745) -> (33.9733, 29.2229) centre (33.9655, 29.1987) ccw
  line L337 (55.633, 1.3208) -> (55.633, 2.4892)
  arc A1073 (26.6305, 29.6644) -> (26.5797, 29.6644) centre (26.6051, 29.6644) ccw
  arc A1074 (50.9947, 29.8986) -> (50.9947, 29.9494) centre (50.9947, 29.924) ccw
  arc A1075 (55.6584, 2.4892) -> (55.6076, 2.4892) centre (55.633, 2.4892) ccw
  arc A1076 (58.9788, 10.1219) -> (59.0296, 10.1219) centre (59.0042, 10.1219) ccw
  arc A1077 (59.1253, 11.1916) -> (59.1427, 11.2394) centre (59.134, 11.2155) ccw
  arc A1078 (57.8499, 14.0955) -> (57.8217, 14.0533) centre (57.8358, 14.0744) ccw
  arc A1079 (59.0156, 12.8511) -> (58.9928, 12.8966) centre (59.0042, 12.8739) ccw
  arc A1080 (58.9901, 13.2743) -> (59.0183, 13.3166) centre (59.0042, 13.2954) ccw
  arc A1081 (36.679, 1.2954) -> (36.679, 1.3462) centre (36.679, 1.3208) ccw
  arc A1082 (57.8217, 13.3166) -> (57.8499, 13.2743) centre (57.8358, 13.2954) ccw
  arc A1083 (60.3758, 8.9662) -> (60.3758, 8.9154) centre (60.3758, 8.9408) ccw
  arc A1084 (60.7004, 9.5899) -> (60.3758, 9.2654) centre (60.7004, 9.2653) ccw
  arc A1085 (58.5103, 12.5493) -> (58.4595, 12.5493) centre (58.4849, 12.5493) ccw
  arc A1086 (57.8104, 12.2248) -> (57.8612, 12.2248) centre (57.8358, 12.2248) ccw
  line L338 (54.6885, 2.4892) -> (54.9481, 2.4892)
  arc A1087 (57.8104, 12.5493) -> (57.8612, 12.5493) centre (57.8358, 12.5493) ccw
  line L339 (58.4849, 12.5493) -> (58.4849, 12.2248)
  line L340 (59.0042, 12.2248) -> (57.8358, 12.2248)
  line L341 (61.5442, 8.9408) -> (60.3758, 8.9408)
  arc A1088 (60.7004, 9.5645) -> (60.7004, 9.6153) centre (60.7004, 9.5899) ccw
  arc A1089 (54.6885, 1.2954) -> (54.6885, 1.3462) centre (54.6885, 1.3208) ccw
  arc A1090 (53.4819, 1.9953) -> (53.4819, 1.9445) centre (53.4819, 1.9699) ccw
  arc A1091 (60.3504, 9.2654) -> (60.4012, 9.2654) centre (60.3758, 9.2654) ccw
  line L342 (60.7004, 9.5899) -> (61.2196, 9.5899)
  arc A1092 (60.3504, 8.9408) -> (60.4012, 8.9408) centre (60.3758, 8.9408) ccw
  arc A1093 (50.9947, 29.924) -> (50.7351, 29.6644) centre (50.9947, 29.6644) ccw
  arc A1094 (59.0042, 12.1994) -> (59.0042, 12.2502) centre (59.0042, 12.2248) ccw
  arc A1095 (54.4034, 2.2296) -> (54.4542, 2.2296) centre (54.4288, 2.2296) ccw
  arc A1096 (34.2067, 29.7329) -> (34.2435, 29.768) centre (34.2251, 29.7505) ccw
  arc A1097 (58.4849, 12.5493) -> (57.8358, 12.5493) centre (58.1604, 12.5493) ccw
  arc A1098 (26.5797, 29.6644) -> (26.6305, 29.6644) centre (26.6051, 29.6644) ccw
  arc A1099 (61.5188, 9.2654) -> (61.5696, 9.2654) centre (61.5442, 9.2654) ccw
  arc A1100 (36.3798, 2.4892) -> (36.329, 2.4892) centre (36.3544, 2.4892) ccw
  arc A1101 (60.7004, 9.6153) -> (60.7004, 9.5645) centre (60.7004, 9.5899) ccw
  arc A1102 (60.5492, 10.2421) -> (60.5269, 10.1964) centre (60.5381, 10.2192) ccw
  arc A1103 (60.4012, 9.2654) -> (60.3504, 9.2654) centre (60.3758, 9.2654) ccw
  arc A1104 (61.2196, 9.5645) -> (61.2196, 9.6153) centre (61.2196, 9.5899) ccw
  line L343 (57.8358, 12.2248) -> (57.8358, 12.5493)
  arc A1105 (57.8612, 12.5493) -> (57.8104, 12.5493) centre (57.8358, 12.5493) ccw
  line L344 (59.0042, 12.8739) -> (58.4849, 12.6142)
  arc A1106 (33.6978, 28.4044) -> (33.7138, 28.3562) centre (33.7058, 28.3803) ccw
  line L345 (61.5442, 9.2654) -> (61.5442, 8.9408)
  arc A1107 (33.9979, 29.8224) -> (33.9979, 29.8732) centre (33.9979, 29.8478) ccw
  line L346 (60.3758, 8.9408) -> (60.3758, 9.2654)
  arc A1108 (33.7312, 29.5557) -> (33.6804, 29.5557) centre (33.7058, 29.5557) ccw
  arc A1109 (61.5442, 8.9154) -> (61.5442, 8.9662) centre (61.5442, 8.9408) ccw
  arc A1110 (34.2251, 29.7505) -> (33.9979, 29.8478) centre (33.998, 29.5341) ccw
  arc A1111 (33.7058, 29.5557) -> (33.9654, 29.1987) centre (34.081, 29.5557) ccw
  line L347 (57.8358, 13.2955) -> (59.0042, 14.0744)
  arc A1112 (61.5188, 8.9408) -> (61.5696, 8.9408) centre (61.5442, 8.9408) ccw
  arc A1113 (57.7147, 11.7587) -> (57.6973, 11.7109) centre (57.706, 11.7348) ccw
  arc A1114 (58.4595, 12.5493) -> (58.5103, 12.5493) centre (58.4849, 12.5493) ccw
  arc A1115 (58.4736, 12.6369) -> (58.4963, 12.5915) centre (58.4849, 12.6142) ccw
  arc A1116 (61.5442, 9.2654) -> (61.2196, 9.5899) centre (61.2196, 9.2653) ccw
  arc A1117 (59.0296, 10.771) -> (58.9788, 10.771) centre (59.0042, 10.771) ccw
  arc A1118 (58.4595, 12.2248) -> (58.5103, 12.2248) centre (58.4849, 12.2248) ccw
  line L348 (59.0042, 13.2955) -> (57.8358, 14.0744)
  arc A1119 (57.8358, 12.2502) -> (57.8358, 12.1994) centre (57.8358, 12.2248) ccw
  arc A1120 (59.0183, 14.0533) -> (58.9901, 14.0955) centre (59.0042, 14.0744) ccw
  arc A1121 (61.2196, 9.6153) -> (61.2196, 9.5645) centre (61.2196, 9.5899) ccw
  arc A1122 (60.3504, 10.4464) -> (60.4012, 10.4465) centre (60.3758, 10.4465) ccw
  arc A1123 (61.3737, 10.2433) -> (61.3902, 10.1952) centre (61.382, 10.2192) ccw
  arc A1124 (60.3504, 12.1031) -> (60.4012, 12.1031) centre (60.3758, 12.1031) ccw
  arc A1125 (61.5301, 13.0838) -> (61.5583, 13.1261) centre (61.5442, 13.105) ccw
  arc A1126 (43.4975, 9.6224) -> (43.4467, 9.6224) centre (43.4721, 9.6224) ccw
  arc A1127 (61.5696, 10.4464) -> (61.5188, 10.4465) centre (61.5442, 10.4465) ccw
  arc A1128 (60.6513, 10.7259) -> (60.6196, 10.6863) centre (60.6354, 10.7061) ccw
  arc A1129 (60.2547, 11.7587) -> (60.2373, 11.7109) centre (60.246, 11.7348) ccw
  arc A1130 (60.4012, 12.7522) -> (60.3504, 12.7522) centre (60.3758, 12.7522) ccw
  line L349 (60.3758, 13.105) -> (61.5442, 13.8839)
  arc A1131 (42.6212, 10.4733) -> (42.5704, 10.4733) centre (42.5958, 10.4733) ccw
  line L350 (61.5442, 13.105) -> (60.3758, 13.8839)
  arc A1132 (61.3931, 10.1964) -> (61.3708, 10.2421) centre (61.382, 10.2192) ccw
  arc A1133 (60.96, 10.7456) -> (60.96, 10.7964) centre (60.96, 10.771) ccw
  arc A1134 (60.5381, 10.2193) -> (60.96, 10.1219) centre (60.9601, 11.0846) ccw
  arc A1135 (60.96, 10.0965) -> (60.96, 10.1473) centre (60.96, 10.1219) ccw
  arc A1136 (61.6653, 11.1916) -> (61.6827, 11.2394) centre (61.674, 11.2155) ccw
  arc A1137 (61.3708, 10.6508) -> (61.3931, 10.6965) centre (61.382, 10.6737) ccw
  line L351 (61.5442, 12.4276) -> (60.3758, 12.4276)
  arc A1138 (61.5583, 13.8628) -> (61.5301, 13.905) centre (61.5442, 13.8839) ccw
  arc A1139 (60.5381, 10.6736) -> (60.3758, 10.4465) centre (60.6159, 10.4465) ccw
  arc A1140 (60.3617, 13.1261) -> (60.3899, 13.0838) centre (60.3758, 13.1049) ccw
  line L352 (43.4721, 9.6224) -> (43.4721, 9.0382)
  arc A1141 (60.3758, 10.4465) -> (60.5381, 10.2193) centre (60.616, 10.4465) ccw
  arc A1142 (43.7722, 9.6956) -> (43.7562, 9.7438) centre (43.7642, 9.7197) ccw
  arc A1143 (42.5878, 9.3544) -> (42.6038, 9.3062) centre (42.5958, 9.3303) ccw
  arc A1144 (60.5463, 10.6496) -> (60.5298, 10.6977) centre (60.5381, 10.6737) ccw
  arc A1145 (61.5442, 10.4465) -> (61.3819, 10.6736) centre (61.3041, 10.4465) ccw
  arc A1146 (42.7692, 10.2689) -> (42.7469, 10.2232) centre (42.758, 10.246) ccw
  arc A1147 (42.7581, 10.7005) -> (42.5958, 10.4733) centre (42.836, 10.4733) ccw
  arc A1148 (43.18, 10.7978) -> (42.7581, 10.7005) centre (43.1798, 9.8351) ccw
  arc A1149 (60.96, 10.1219) -> (61.3819, 10.2193) centre (60.9599, 11.0846) ccw
  arc A1150 (61.5696, 9.2654) -> (61.5188, 9.2654) centre (61.5442, 9.2654) ccw
  arc A1151 (60.96, 10.1473) -> (60.96, 10.0965) centre (60.96, 10.1219) ccw
  arc A1152 (60.3899, 13.905) -> (60.3617, 13.8628) centre (60.3758, 13.8839) ccw
  arc A1153 (60.96, 10.7964) -> (60.96, 10.7456) centre (60.96, 10.771) ccw
  line L353 (42.5958, 9.3303) -> (43.7642, 9.7197)
  arc A1154 (60.3758, 12.453) -> (60.3758, 12.4022) centre (60.3758, 12.4276) ccw
  arc A1155 (42.5958, 10.4733) -> (42.7581, 10.2461) centre (42.836, 10.4733) ccw
  arc A1156 (61.3819, 10.6736) -> (60.96, 10.771) centre (60.9599, 9.8083) ccw
  arc A1157 (42.6038, 9.3544) -> (42.5878, 9.3062) centre (42.5958, 9.3303) ccw
  arc A1158 (61.3902, 10.6977) -> (61.3737, 10.6496) centre (61.382, 10.6737) ccw
  arc A1159 (42.5704, 10.4733) -> (42.6212, 10.4733) centre (42.5958, 10.4733) ccw
  arc A1160 (42.7469, 10.7233) -> (42.7692, 10.6776) centre (42.758, 10.7005) ccw
  arc A1161 (61.5188, 10.4464) -> (61.5696, 10.4465) centre (61.5442, 10.4465) ccw
  arc A1162 (42.7581, 10.2461) -> (43.18, 10.1487) centre (43.1801, 11.1114) ccw
  arc A1163 (60.5269, 10.6965) -> (60.5492, 10.6508) centre (60.5381, 10.6737) ccw
  arc A1164 (61.2687, 10.167) -> (61.3004, 10.2066) centre (61.2846, 10.1868) ccw
  line L354 (61.2846, 10.1868) -> (60.6354, 10.7061)
  arc A1165 (60.96, 10.771) -> (60.5381, 10.6736) centre (60.9601, 9.8083) ccw
  arc A1166 (61.5442, 12.4022) -> (61.5442, 12.453) centre (61.5442, 12.4276) ccw
  line L355 (60.3758, 12.1031) -> (60.3758, 12.7522)
  arc A1167 (60.4012, 10.4464) -> (60.3504, 10.4465) centre (60.3758, 10.4465) ccw
  line L356 (43.7642, 8.9408) -> (42.5958, 9.3303)
  arc A1168 (60.5298, 10.1952) -> (60.5463, 10.2433) centre (60.5381, 10.2193) ccw
  arc A1169 (43.7562, 8.9167) -> (43.7722, 8.9649) centre (43.7642, 8.9408) ccw
  arc A1170 (43.4467, 9.0382) -> (43.4975, 9.0382) centre (43.4721, 9.0382) ccw
  arc A1171 (42.7498, 10.222) -> (42.7663, 10.2701) centre (42.758, 10.2461) ccw
  arc A1172 (43.18, 10.1233) -> (43.18, 10.1741) centre (43.18, 10.1487) ccw
  line L357 (61.674, 11.2155) -> (60.246, 11.7348)
  arc A1173 (42.7663, 10.6764) -> (42.7498, 10.7245) centre (42.758, 10.7005) ccw
  arc A1174 (43.18, 10.1741) -> (43.18, 10.1233) centre (43.18, 10.1487) ccw
  arc A1175 (61.3819, 10.2193) -> (61.5442, 10.4465) centre (61.304, 10.4465) ccw
  arc A1176 (43.6131, 10.2232) -> (43.5908, 10.2689) centre (43.602, 10.2461) ccw
  arc A1177 (43.18, 10.1487) -> (43.6019, 10.2461) centre (43.1799, 11.1114) ccw
  arc A1178 (43.6019, 10.2461) -> (43.7642, 10.4733) centre (43.524, 10.4733) ccw
  arc A1179 (43.7388, 10.4733) -> (43.7896, 10.4733) centre (43.7642, 10.4733) ccw
  line L358 (55.9774, 12.6873) -> (55.7826, 12.3303)
  arc A1180 (56.4896, 13.7889) -> (56.4388, 13.7889) centre (56.4642, 13.7889) ccw
  arc A1181 (45.1358, 10.4987) -> (45.1358, 10.4479) centre (45.1358, 10.4733) ccw
  arc A1182 (55.4135, 12.737) -> (55.3728, 12.7674) centre (55.3932, 12.7522) ccw
  arc A1183 (45.1278, 9.3544) -> (45.1438, 9.3062) centre (45.1358, 9.3303) ccw
  arc A1184 (42.8713, 10.7527) -> (42.8396, 10.7131) centre (42.8554, 10.7329) ccw
  arc A1185 (45.1556, 10.4891) -> (45.116, 10.4574) centre (45.1358, 10.4732) ccw
  line L359 (45.3954, 10.1487) -> (45.1358, 10.4733)
  arc A1186 (43.18, 10.8232) -> (43.18, 10.7724) centre (43.18, 10.7978) ccw
  arc A1187 (46.2962, 8.9167) -> (46.3122, 8.9649) centre (46.3042, 8.9408) ccw
  line L360 (45.1358, 9.3303) -> (46.3042, 9.7197)
  line L361 (46.3042, 10.1487) -> (46.3042, 10.7978)
  arc A1188 (48.8522, 9.6956) -> (48.8362, 9.7438) centre (48.8442, 9.7197) ccw
  arc A1189 (56.4388, 13.5292) -> (56.4896, 13.5292) centre (56.4642, 13.5292) ccw
  arc A1190 (48.8362, 8.9167) -> (48.8522, 8.9649) centre (48.8442, 8.9408) ccw
  arc A1191 (47.6838, 9.3544) -> (47.6678, 9.3062) centre (47.6758, 9.3303) ccw
  arc A1192 (48.5775, 9.6224) -> (48.5267, 9.6224) centre (48.5521, 9.6224) ccw
  arc A1193 (56.2046, 13.2696) -> (56.4642, 13.5292) centre (56.2046, 13.5292) ccw
  arc A1194 (56.2046, 13.295) -> (56.2046, 13.2442) centre (56.2046, 13.2696) ccw
  arc A1195 (46.3122, 9.6956) -> (46.2962, 9.7438) centre (46.3042, 9.7197) ccw
  arc A1196 (45.3756, 10.1328) -> (45.4153, 10.1646) centre (45.3955, 10.1487) ccw
  line L362 (43.5046, 10.2136) -> (42.8554, 10.7329)
  arc A1197 (43.5937, 10.2701) -> (43.6102, 10.222) centre (43.602, 10.246) ccw
  arc A1198 (43.7642, 10.4733) -> (43.6019, 10.7005) centre (43.524, 10.4733) ccw
  line L363 (46.3042, 8.9408) -> (45.1358, 9.3303)
  arc A1199 (43.4887, 10.1938) -> (43.5204, 10.2335) centre (43.5045, 10.2137) ccw
  arc A1200 (54.6885, 2.4892) -> (54.4288, 2.2296) centre (54.6885, 2.2295) ccw
  arc A1201 (46.2788, 10.1487) -> (46.3296, 10.1487) centre (46.3042, 10.1487) ccw
  arc A1202 (56.2046, 12.8171) -> (55.9774, 12.6873) centre (56.2046, 12.5534) ccw
  line L364 (56.4642, 13.7889) -> (56.4642, 13.5292)
  arc A1203 (46.3296, 10.7978) -> (46.2788, 10.7978) centre (46.3042, 10.7978) ccw
  line L365 (47.6758, 9.3303) -> (48.8442, 9.7197)
  arc A1204 (45.9867, 9.0382) -> (46.0375, 9.0382) centre (46.0121, 9.0382) ccw
  line L366 (48.8442, 8.9408) -> (47.6758, 9.3303)
  arc A1205 (43.7896, 10.4733) -> (43.7388, 10.4733) centre (43.7642, 10.4733) ccw
  line L367 (27.2542, 30.7425) -> (26.0858, 31.1319)
  arc A1206 (43.5908, 10.6776) -> (43.6131, 10.7233) centre (43.602, 10.7005) ccw
  arc A1207 (43.6019, 10.7005) -> (43.18, 10.7978) centre (43.1802, 9.8351) ccw
  arc A1208 (43.6102, 10.7245) -> (43.5937, 10.6764) centre (43.602, 10.7005) ccw
  line L368 (46.0121, 9.6224) -> (46.0121, 9.0382)
  arc A1209 (45.1438, 9.3544) -> (45.1278, 9.3062) centre (45.1358, 9.3303) ccw
  arc A1210 (46.3042, 10.4479) -> (46.3042, 10.4987) centre (46.3042, 10.4733) ccw
  arc A1211 (47.6678, 9.3544) -> (47.6838, 9.3062) centre (47.6758, 9.3303) ccw
  arc A1212 (47.9679, 10.7978) -> (47.6758, 10.5057) centre (47.9679, 10.5057) ccw
  arc A1213 (26.8647, 29.9494) -> (26.8647, 29.8986) centre (26.8647, 29.924) ccw
  arc A1214 (55.2704, 12.4601) -> (55.3212, 12.4601) centre (55.2958, 12.4601) ccw
  arc A1215 (55.8045, 12.3174) -> (55.7608, 12.3432) centre (55.7827, 12.3303) ccw
  arc A1216 (46.0375, 9.6224) -> (45.9867, 9.6224) centre (46.0121, 9.6224) ccw
  line L369 (48.5521, 9.6224) -> (48.5521, 9.0382)
  arc A1217 (26.6051, 29.2495) -> (26.6051, 29.3003) centre (26.6051, 29.2749) ccw
  arc A1218 (29.7688, 28.2504) -> (29.8196, 28.2504) centre (29.7942, 28.2504) ccw
  arc A1219 (55.9997, 12.6751) -> (55.9551, 12.6995) centre (55.9774, 12.6873) ccw
  arc A1220 (56.2046, 12.7917) -> (56.2046, 12.8425) centre (56.2046, 12.8171) ccw
  arc A1221 (48.5267, 9.0382) -> (48.5775, 9.0382) centre (48.5521, 9.0382) ccw
  arc A1222 (43.18, 10.7724) -> (43.18, 10.8232) centre (43.18, 10.7978) ccw
  line L370 (45.1358, 10.4733) -> (46.3042, 10.4733)
  arc A1223 (55.9555, 12.7002) -> (55.9993, 12.6744) centre (55.9774, 12.6873) ccw
  arc A1224 (55.5554, 12.2005) -> (55.7826, 12.3303) centre (55.5554, 12.4642) ccw
  arc A1225 (55.5554, 12.2259) -> (55.5554, 12.1751) centre (55.5554, 12.2005) ccw
  arc A1226 (55.7603, 12.3424) -> (55.8049, 12.3181) centre (55.7826, 12.3302) ccw
  arc A1227 (56.4896, 13.5292) -> (56.4388, 13.5292) centre (56.4642, 13.5292) ccw
  arc A1228 (35.7547, 10.8486) -> (35.7547, 10.8994) centre (35.7547, 10.874) ccw
  arc A1229 (35.6644, 8.9408) -> (35.7152, 8.9408) centre (35.6898, 8.9408) ccw
  line L371 (33.5393, 9.3303) -> (32.7604, 9.3303)
  arc A1230 (33.1244, 8.9408) -> (33.1752, 8.9408) centre (33.1498, 8.9408) ccw
  line L372 (33.6042, 11.6925) -> (32.4358, 12.0819)
  arc A1231 (32.9297, 10.2249) -> (32.9805, 10.2249) centre (32.9551, 10.2249) ccw
  line L373 (33.6042, 10.2249) -> (33.6042, 10.6144)
  arc A1232 (55.3212, 13.5292) -> (55.2704, 13.5292) centre (55.2958, 13.5292) ccw
  arc A1233 (35.3004, 9.3557) -> (35.3004, 9.3049) centre (35.3004, 9.3303) ccw
  arc A1234 (33.1752, 9.7197) -> (33.1244, 9.7197) centre (33.1498, 9.7197) ccw
  line L374 (32.9551, 10.6144) -> (32.9551, 10.2249)
  arc A1235 (55.2704, 13.5292) -> (55.3212, 13.5292) centre (55.2958, 13.5292) ccw
  arc A1236 (56.4642, 14.2404) -> (56.4642, 14.2912) centre (56.4642, 14.2658) ccw
  arc A1237 (56.4896, 14.7851) -> (56.4388, 14.7851) centre (56.4642, 14.7851) ccw
  arc A1238 (56.2046, 13.2442) -> (56.2046, 13.295) centre (56.2046, 13.2696) ccw
  line L375 (56.2046, 13.2696) -> (55.5554, 13.2696)
  arc A1239 (56.4388, 14.2658) -> (56.4896, 14.2658) centre (56.4642, 14.2658) ccw
  arc A1240 (32.9551, 10.1995) -> (32.9551, 10.2503) centre (32.9551, 10.2249) ccw
  line L376 (56.4642, 14.2658) -> (56.4642, 14.7851)
  arc A1241 (32.4438, 12.106) -> (32.4278, 12.0578) centre (32.4358, 12.0819) ccw
  line L377 (36.0793, 9.3303) -> (35.3004, 9.3303)
  line L378 (36.1442, 10.2249) -> (36.1442, 10.6144)
  arc A1242 (36.1696, 10.6144) -> (36.1188, 10.6144) centre (36.1442, 10.6144) ccw
  line L379 (35.8846, 10.874) -> (35.7547, 10.874)
  line L380 (33.1498, 8.9408) -> (33.1498, 9.7197)
  arc A1243 (33.5788, 10.2249) -> (33.6296, 10.2249) centre (33.6042, 10.2249) ccw